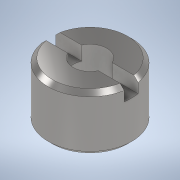
# Autodesk Inventor part: ARU-304S
Saved by Autodesk Inventor 2020 (Build 240168000, 168)
## iProperties
Created: 2021-09-06
Part Number: ARU-304S
Material: ステンレス鋼 440C
Document SubType Name: Modeling
Designer: Masato
Density: 7.75 g/cm^3
Appearance: 半つや出し
Mass: 0.880084 g
Surface Area: 1.76155 cm^2
Volume: 0.113559 cm^3
Author: Masato
Autodesk Inventor part; units mm, degrees
ref_plane "YZ Plane" through (0, 0, 0) normal (1, 0, 0) x (0, 1, 0)
ref_plane "XZ Plane" through (0, 0, 0) normal (0, 1, 0) x (-1, 0, 0)
ref_plane "XY Plane" through (0, 0, 0) normal (0, 0, 1) x (1, 0, 0)
sketch "スケッチ1" plane through (0, 0, 0) normal (0, 0, 1) x (1, 0, 0)
  line L0 (1.2, -2) -> (1.2, 2)
  line L1 (1.2, 2) -> (2.7, 2)
  line L2 (2.7, 2) -> (3, 1.7)
  line L3 (3, 1.7) -> (3, -1.7)
  line L4 (0, 6.4765) -> (0, -6.4765) construction
  line L5 (3, -1.7) -> (2.7, -2)
  line L6 (2.7, -2) -> (1.2, -2)
  point P0 (0, 0)
  point P1 (0, 0)
  point P2 (0, 0)
  point P3 (1.2, 0)
  point P4 (3, 0)
  dimension "d0" = 6
  dimension "d1" = 2.4
  dimension "d2" = 4
  dimension "d3" = 0.3
  dimension "d4" = 0.3
  constraints: 14 end point, 3 midpoint, 2 coincident, 2 horizontal alignment, 2 perpendicular, 1 horizontal, 1 parallel, 1 vertical
  measures "d0" diameter of L3 L4
  measures "d1" diameter of L0 L4
  measures "d2" distance between parallel lines of L6 L1
  measures "d3" horizontal distance of L2.end L1.end
  measures "d4" horizontal distance of L1.end L2.end
revolve "回転1" add sketch "スケッチ1" angle 360 about axis through (0, 6.4765, 0) along (0, -1, 0)
sketch "スケッチ2" plane through (0, 2, 0) normal (0, 1, 0) x (1, 0, 0)
  line L0 (-3, -0.5) -> (3, -0.5)
  line L1 (3, -0.5) -> (3, 0.5)
  line L2 (3, 0.5) -> (-3, 0.5)
  line L3 (-3, 0.5) -> (-3, -0.5)
  line L4 (-3, -0.5) -> (3, 0.5) construction
  line L5 (3, -0.5) -> (-3, 0.5) construction
  circle A0 centre (0, 0) radius 3 projected
  point P0 (0, 0)
  point P1 (2.958, -0.5)
  point P2 (2.958, 0.5)
  point P3 (-2.958, 0.5)
  point P4 (-2.958, -0.5)
  dimension "d6" = 1
  constraints: 12 end point, 2 midpoint, 2 parallel, 1 horizontal, 1 perpendicular, 1 tangent
  measures "d6" distance of L1.end L0.end
extrude "押し出し1" cut sketch "スケッチ2" against normal blind 1 contours A0 L2 L0
equation "\"d4\" = d3"
